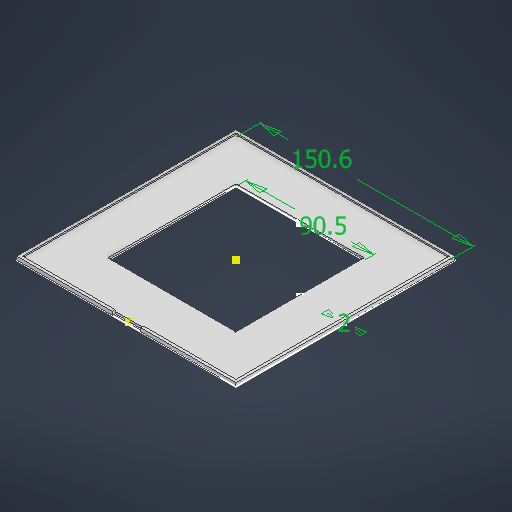
# Autodesk Inventor part: 15cmPasteMaskTemplate
Saved by Autodesk Inventor 2026 (Build 300175050, 175E)
## iProperties
Created: 2025-07-24
Part Number: 15cmPasteMaskTemplate
Material: Generic
Document SubType Name: Modeling
Designer: user
Density: 1 g/cm^3
Appearance: Default
Author: user
## iProperties of the stored document 15cmPasteMaskTemplate_3DPrint.ipt
Created: 2025-07-24
Part Number: 15cmPasteMaskTemplate_3DPrint
Material: Generic
Document SubType Name: Modeling
Designer: user
Density: 1 g/cm^3
Appearance: Default
Author: user
Autodesk Inventor part; units mm, degrees
ref_plane "YZ Plane" through (0, 0, 0) normal (1, 0, 0) x (0, 1, 0)
ref_plane "XZ Plane" through (0, 0, 0) normal (0, 1, 0) x (-1, 0, 0)
ref_plane "XY Plane" through (0, 0, 0) normal (0, 0, 1) x (1, 0, 0)
sketch "Sketch1" plane through (0, 0, 0) normal (0, 1, 0) x (-1, 0, 0)
  line L0 (45.25, -45.25) -> (-45.25, -45.25)
  line L1 (-45.25, -45.25) -> (-45.25, 45.25)
  line L2 (-45.25, 45.25) -> (45.25, 45.25)
  line L3 (45.25, 45.25) -> (45.25, -45.25)
  line L4 (75.3, -75.3) -> (-75.3, -75.3)
  line L5 (-75.3, -75.3) -> (-75.3, 75.3)
  line L6 (-75.3, 75.3) -> (75.3, 75.3)
  line L7 (75.3, 75.3) -> (75.3, -75.3)
  line L8 (-77.3, 77.3) -> (-77.3, -77.3)
  line L9 (-77.3, -77.3) -> (77.3, -77.3)
  line L10 (77.3, -77.3) -> (77.3, 77.3)
  line L11 (77.3, 77.3) -> (-77.3, 77.3)
  point P0 (0, 0)
  point P1 (-45.25, 0)
  point P2 (0, -45.25)
  point P3 (-75.3, 0)
  point P4 (0, -75.3)
  dimension "d0" = 90.5
  dimension "d1" = 150.6
  dimension "d2" = 2
  constraints: 24 end point, 6 parallel, 5 perpendicular, 4 midpoint, 2 horizontal, 2 horizontal alignment, 2 vertical alignment, 3 other
  measures "d0" distance of L0.start L0.end
  measures "d1" distance of L4.start L4.end
  measures "d2" distance between parallel lines of L5 L8
extrude "Extrusion1" add sketch "Sketch1" along normal blind 1.5 contours L4 L5 L6 L7
extrude "Extrusion2" add sketch "Sketch1" along normal blind 2.5 contours L11 L10 L9 L8
sketch "Sketch2" plane through (75.3, 1.5, 75.3) normal (0, 0, -1) x (-1, 0, 0)
  point P0 (75.3, -1.5)
sketch "Sketch3" plane through (-77.3, 0, 77.3) normal (0, 0, 1) x (1, 0, 0)
  line L0 (152.6, 2.5) -> (2, 2.5) projected
  line L1 (67.3, 2.5) -> (87.3, 2.5)
  line L2 (87.3, 2.5) -> (87.3, 0)
  line L3 (87.3, 0) -> (67.3, 0)
  line L4 (67.3, 0) -> (67.3, 2.5)
  line L5 (0, 0) -> (154.6, 0) projected
  line L6 (2, 1.5) -> (152.6, 1.5) projected
  line L7 (152.6, 1.5) -> (2, 1.5) projected
  line L8 (32.05, 1.5) -> (122.55, 1.5) projected
  line L9 (122.55, 1.5) -> (32.05, 1.5) projected
  point P0 (77.3, 0)
  point P1 (77.3, 0)
  point P2 (77.3, 0)
  dimension "d7" = 20
  constraints: 8 end point, 2 midpoint, 2 parallel, 1 coincident, 1 collinear, 1 horizontal, 1 perpendicular, 1 point on line
  measures "d7" distance of L2.end L3.end
extrude "Extrusion3" cut sketch "Sketch3" against normal up to surface (2 mm away)
body "Solid1"
